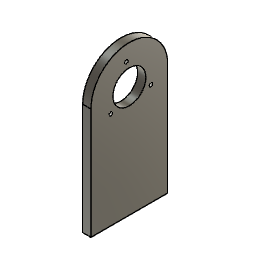
Bika Chassis Design (Autodesk Fusion 360 archive; units mm, degrees)
design "Reaction Wheel Holder"
Autodesk Fusion 360 part; units mm, degrees
sketch "sketch" plane through (0, 0, 0) normal (1, 0, 0) x (0, 1, 0)
  arc A0 (28, 0) -> (-28, 0) centre (0, 0) ccw
  line L0 (-28, -81) -> (28, -81)
  circle A1 centre (0, 0) radius 12
  line L1 (28, -81) -> (28, 0)
  line L2 (-28, 0) -> (-28, -81)
  circle A2 centre (-2.1649, 16.8616) radius 1.6
  circle A3 centre (-13.5201, -10.3057) radius 1.6
  circle A4 centre (15.685, -6.5559) radius 1.6
  dimension "d8" = 3.2
  measures "d8" diameter of A2
extrude "Extrude1" add sketch "sketch" along normal blind 6
thread "Thread1" "ISO Metric profile 3.0 M3x0.5 6H" major diameter 3.086 minor diameter 2.529 pitch 0.5 angle 60 resizes the face on face at (4, 17.283, -6.6357)
thread "Thread2" "ISO Metric profile 3.0 M3x0.5 6H" major diameter 3.086 minor diameter 2.529 pitch 0.5 angle 60 resizes the face on face at (2, -0.5669, 16.9413)
thread "Thread3" "ISO Metric profile 3.0 M3x0.5 6H" major diameter 3.086 minor diameter 2.529 pitch 0.5 angle 60 resizes the face on face at (4, -11.928, -10.1464)
sketch "Sketch2" plane through (6, 0, 0) normal (1, 0, 0) x (0, 1, 0)
  line L0 (-28, -81) -> (28, -81)
  circle A0 centre (0, 0) radius 12
  circle A1 centre (-13.5201, -10.3057) radius 1.2645
  circle A2 centre (-2.1649, 16.8616) radius 1.2645
  circle A3 centre (15.685, -6.5559) radius 1.2645
  line L1 (-28, -71) -> (26.2723, -71)
  line L2 (26.2723, -71) -> (26.2723, -81)
  line L3 (26.2723, -81) -> (-28, -81)
  line L4 (-28, -71) -> (-44.008, -71)
  line L5 (-44.008, -71) -> (-44.008, -81)
  line L6 (-44.008, -81) -> (-28, -81)
  line L7 (-28, 0) -> (-28, -81)
  line L8 (28, -81) -> (28, 0)
  arc A4 (28, 0) -> (-28, 0) centre (0, 0) ccw
  dimension "d11" = 10
  constraint coincident L0.start L3.end
  constraint perpendicular L0 L2
  constraint perpendicular L0 L5
  measures "d11" distance of L0.start L1.start
extrude "Extrude2" cut sketch "Sketch2" against normal blind 55 contours L0 L1 L2 L3 L7 | L4 L5 L6 L7
extrude "Extrude3" cut 1 faces at (4, -9.9092, -71) along direction (0, 0, 1) blind 7
ref_plane "WorkPlane1" through (3.1597, 0, 28) normal (0, 0, 1) x (0, 1, 0)
extrude "Extrude4" add 1 faces at (4, -9.9092, -64) along direction (0, 0, -1) up to surface (17 mm away)
